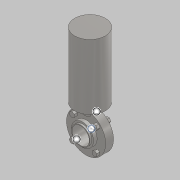
# Autodesk Inventor part: MANUAL SANITARY BUTTERFLY VALVE 304L DN50
Saved by Autodesk Inventor 2017 (Build 210142000, 142)
## iProperties
Category: Plant Design Equipment
Company: Pocket Brewery Belgium
Created: 2017-11-25
Part Number: MANUAL SANITARY BUTTERFLY VALVE 304L DN50
Material: 304L
Document SubType Name: Modeling
Designer: Demarec
Density: 8 g/cm^3
Appearance: Semi-Polished(1)
Catalog Web Link: http://www.pocketbrewery.com
Author: Marc Crauwels
Title: Valves
Comments: This Valve is generated with the Pocket Brewery Valve App. This software is part of the Pocket Brewery Design Suite.
Autodesk Inventor part; units mm, degrees
ref_plane "YZ Plane" through (0, 0, 0) normal (1, 0, 0) x (0, 1, 0)
ref_plane "XZ Plane" through (0, 0, 0) normal (0, 1, 0) x (-1, 0, 0)
ref_plane "XY Plane" through (0, 0, 0) normal (0, 0, 1) x (1, 0, 0)
sketch "Sketch11" plane through (0, 0, 0) normal (0, 1, 0) x (-1, 0, 0)
  circle A0 centre (0, 0) radius 26
  circle A1 centre (0, 0) radius 24
  circle A2 centre (0, 0) radius 31
  circle A3 centre (0, 0) radius 55
  line L0 (35.5726, 38.3198) -> (39.3254, 31.8198)
  line L1 (39.3254, 31.8198) -> (35.5726, 25.3198)
  line L2 (35.5726, 25.3198) -> (28.067, 25.3198)
  line L3 (28.067, 25.3198) -> (24.3143, 31.8198)
  line L4 (24.3143, 31.8198) -> (28.067, 38.3198)
  line L5 (28.067, 38.3198) -> (35.5726, 38.3198)
  line L6 (0, 0) -> (31.8198, 31.8198) construction
  line L7 (0, 0) -> (45, 0) construction
  line L8 (35.5726, 38.3198) -> (28.067, 25.3198) construction
  line L9 (28.067, 38.3198) -> (35.5726, 25.3198) construction
  line L10 (39.3254, 31.8198) -> (24.3143, 31.8198) construction
  line L11 (0, 52.6213) -> (0, 85)
  line L12 (0, 85) -> (-16, 85)
  line L13 (-16, 85) -> (-16, 52.6213)
  line L14 (0, 64) -> (0, 58.5)
  line L15 (-16, 52.6213) -> (0, 52.6213)
  line L16 (0, 52.6213) -> (-16, 52.6213)
  line L17 (-16, 52.6213) -> (-16, 44.6213)
  line L18 (-16, 44.6213) -> (0, 44.6213)
  line L19 (0, 44.6213) -> (0, 52.6213)
  line L20 (0, 68.8106) -> (-43, 68.8106)
  line L21 (-43, 68.8106) -> (-43, 250.8106)
  line L22 (-43, 250.8106) -> (0, 250.8106)
  line L23 (0, 250.8106) -> (0, 68.8106)
  dimension "oOuterDia" = 110
  dimension "oPipeDia" = 52
  dimension "oPipeWall" = 2
  dimension "oPipeLenght" = 5
  dimension "oKdia" = 45
  dimension "d70" = 45
  dimension "oSW" = 13
  dimension "oCenterTop" = 85
  dimension "d78" = 16
  dimension "d86" = 8
  dimension "oActuatorDia" = 43
  dimension "oActuatorLenght" = 182
  constraints: 48 end point, 7 equal length, 5 horizontal, 5 parallel, 4 perpendicular, 3 centre point, 2 coincident, 2 midpoint, 2 point on line, 1 vertical, 3 other
  measures "oPipeDia" diameter of A0
  measures "oPipeWall" radial gap between concentric circles of A0 A1
  measures "oPipeLenght" radial gap between concentric circles of A2 A0
  measures "oKdia" distance of L6.end L6.start
  measures "d70" angle of L7 L6
  measures "oSW" distance between parallel lines of L2 L5
  measures "oCenterTop" distance from line of L12 point (0, 0)
  measures "d78" distance of L11.end L12.end
  measures "d86" distance of L13.end L17.end
  measures "oActuatorDia" distance of L21.end L22.end
  measures "oActuatorLenght" distance of L20.end L21.end
extrude "Extrusion12" add sketch "Sketch11" along normal mid plane 52 contours A0
extrude "Extrusion13" add sketch "Sketch11" along normal mid plane 42 contours A2
extrude "Extrusion14" add sketch "Sketch11" along normal mid plane 22 contours L17 L18 L19 L11 A3 | A3 L11 L15 | L15 L19 L18 L17 | L0 L1 L2 L3 L4 L5
extrude "Extrusion15" add sketch "Sketch11" along normal mid plane 38 contours L0 L1 L2 L3 L4 L5
pattern_circular "Circular Pattern2" count 4 over 360 about axis through (0, 0, 0) along (0, 1, 0) of "Extrusion15"
revolve "Revolution1" add sketch "Sketch11" angle 360 about axis through (0, 0, 52.6213) along (0, 0, 1) contours L13 L20 L11 A3 | A3 L11 L15 | L15 L19 L18 L17 | L13 L12 L11 L20
revolve "Revolution4" add sketch "Sketch11" angle 360 about axis through (0, 0, 250.8106) along (0, 0, -1) contours L20 L21 L22 L23 L12 L13 | L13 L12 L11 L20
equation "\"d65\" = -2 * oPipeLenght + oValveLenght"
equation "\"oValveLenght\" = 52"
body "Solid1"
body "Solid2"
